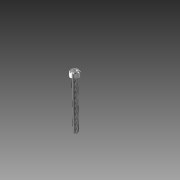
# Autodesk Inventor part: tornillo allen m3x30
Saved by Autodesk Inventor 2012 SP2 (Build 160219200, 219)
## iProperties
Shininess: 64.0
Length Units: 11269
Angle Units: 11279
Time Units: 11290
Mass Units: 11283
Length Display Precision: 4
Angle Display Precision: 2
Compacted: True
Created: 2002-08-23
Part Number: tornillo allen m3x30
Material: Grade 8.8
Description: DIN 912 - M12x30
Document SubType Name: Modeling
Designer: Cor de Vlaming
Engineer: Cor de Vlaming
Density: 7.75 g/cm^3
Density: 0.0
Volumn: 0.0
Area: 0.0
PropertySet Name: Model Information
Control State: 0
Master: False
Checked Out: False
Author: Cor de Vlaming
Autodesk Inventor part; units mm, degrees
ref_plane "YZ Plane" through (0, 0, 0) normal (1, 0, 0) x (0, 1, 0)
ref_plane "XZ Plane" through (0, 0, 0) normal (0, 1, 0) x (-1, 0, 0)
ref_plane "XY Plane" through (0, 0, 0) normal (0, 0, 1) x (1, 0, 0)
sketch "Sketch1" plane through (0, 0, 0) normal (0, 0, 1) x (1, 0, 0)
  circle A0 centre (0, 0) radius 1.5
  dimension "Diameter" = 3
  constraints: 1 centre point
  measures "Diameter" diameter of A0
extrude "Extrusion1" add sketch "Sketch1" along normal blind 30
sketch "Sketch2" plane through (0, 0, 30) normal (0, 0, 1) x (1, 0, 0)
  circle A0 centre (0, 0) radius 1.5 projected
  circle A1 centre (0, 0) radius 2.75
  dimension "Kopdiameter" = 5.5
  constraints: 1 centre point, 1 coincident
  measures "Kopdiameter" diameter of A1
extrude "Extrusion2" add sketch "Sketch2" along normal blind 3 contours A0 | A1
sketch "Sketch3" plane through (0, 0, 33) normal (0, 0, 1) x (1, 0, 0)
  circle A0 centre (0, 0) radius 2.75 projected
  circle A1 centre (0, 0) radius 1.4434 construction
  line L0 (0, 1.4434) -> (1.25, 0.7217)
  line L1 (1.25, -0.7217) -> (1.25, 0.7217)
  line L2 (0, 1.4434) -> (-1.25, 0.7217)
  line L3 (-1.25, -0.7217) -> (-1.25, 0.7217)
  line L4 (-1.25, -0.7217) -> (0, -1.4434)
  line L5 (1.25, -0.7217) -> (0, -1.4434)
  dimension "Binnenzeskant" = 2.5
  constraints: 12 end point, 6 point on circle, 3 equal length, 1 centre point, 1 coincident, 1 parallel, 1 vertical
  measures "Binnenzeskant" distance between parallel lines of L0 L4
extrude "Extrusion3" cut sketch "Sketch3" against normal blind 1.3 contours L0 L1 L5 L4 L3 L2
thread "Thread1" size "M3x0.5" class "4g6g" standard "ISO Metric profile" full length
chamfer "Chaflán2" distance 0.5 angle 45 2 edges at (-2.75, 0, 33) (-1.5, 0, 0)
equation "\"d9\" = Draadlengte"
equation "\"Draadlengte\" = 24.75"
equation "\"Sizes\" = Diameter"
equation "\"Schroefdraad\" = Sizes"
